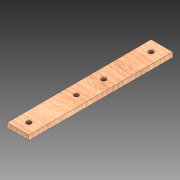
# Autodesk Inventor part: 1211_Distal Roller Plate_V1
Saved by Autodesk Inventor 2020 (Build 240168000, 168)
## iProperties
Created: 2019-09-26
Part Number: 1211_Distal Roller Plate_V1
Material: Wood (Birch)
Document SubType Name: Modeling
Designer: MPI
Density: 0.55 g/cm^3
Appearance: Birch - Natural Polished
Mass: 132.766 g
Surface Area: 344.898 cm^2
Volume: 132.766 cm^3
Author: MPI
Autodesk Inventor part; units mm, degrees
ref_plane "YZ Plane" through (0, 0, 0) normal (1, 0, 0) x (0, 1, 0)
ref_plane "XZ Plane" through (0, 0, 0) normal (0, 1, 0) x (-1, 0, 0)
ref_plane "XY Plane" through (0, 0, 0) normal (0, 0, 1) x (1, 0, 0)
sketch "Sketch1" plane through (0, 0, 0) normal (0, 1, 0) x (-1, 0, 0)
  line L0 (45, 0) -> (0, 0)
  line L1 (0, 0) -> (0, -300)
  line L2 (0, -300) -> (45, -300)
  line L3 (45, -300) -> (45, 0)
  circle A0 centre (22.5, -22.5) radius 5
  circle A1 centre (22.5, -277.5) radius 5
  line L4 (79.2183, -150) -> (-46.459, -150) construction
  circle A2 centre (22.5, -121.5) radius 4.8
  circle A3 centre (22.5, -178.5) radius 4.8
  dimension "d0" = 300
  dimension "d1" = 45
  dimension "d2" = 10
  dimension "d3" = 10
  dimension "d4" = 22.5
  dimension "d5" = 22.5
  dimension "d6" = 22.5
  dimension "d7" = 22.5
  dimension "d8" = 150
  dimension "d9" = 9.6
  dimension "d10" = 28.5
  dimension "d11" = 22.5
  dimension "d12" = 22.5
  dimension "d13" = 28.5
  constraints: 10 end point, 4 centre point, 2 horizontal, 2 parallel, 1 coincident, 1 equal radius, 1 perpendicular
  measures "d0" distance of L2.end L0.start
  measures "d1" distance of L0.start L0.end
  measures "d2" diameter of A0
  measures "d3" diameter of A1
  measures "d4" distance from line of A0.centre L0
  measures "d5" distance from line of L3 A0.centre
  measures "d6" distance from line of L2 A1.centre
  measures "d7" distance from line of A1.centre L3
  measures "d8" distance between parallel lines of L4 L0
  measures "d9" diameter of A2
  measures "d10" distance from line of L4 A2.centre
  measures "d11" distance from line of L3 A3.centre
  measures "d12" distance from line of L3 A2.centre
  measures "d13" distance from line of L4 A3.centre
extrude "Extrusion1" add sketch "Sketch1" along normal blind 10
body "Solid1"
